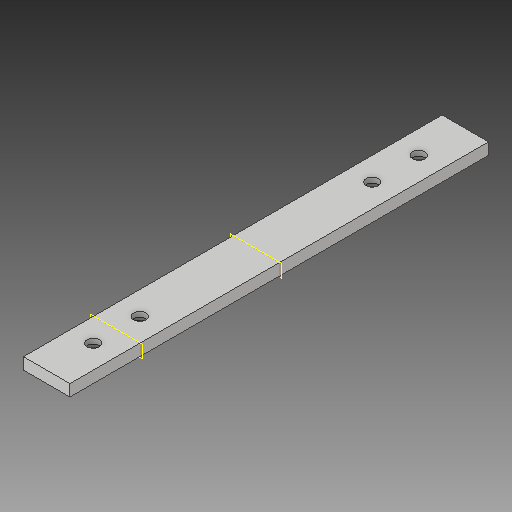
# Autodesk Inventor part: BandSawJigSupport
Saved by Autodesk Inventor 2019 (Build 230136000, 136)
## iProperties
Created: 2017-12-11
Part Number: BandSawJigSupport
Material: Generic
Document SubType Name: Modeling
Designer: steele
Density: 1 g/cm^3
Appearance: Default
Author: steele
Autodesk Inventor part; units mm, degrees
ref_plane "YZ Plane" through (0, 0, 0) normal (1, 0, 0) x (0, 1, 0)
ref_plane "XZ Plane" through (0, 0, 0) normal (0, 1, 0) x (-1, 0, 0)
sketch "Sketch1" plane through (0, 0, 0) normal (0, 1, 0) x (-1, 0, 0)
  line L0 (12.7, 114.3) -> (-12.7, 114.3)
  line L1 (-12.7, 114.3) -> (-12.7, -114.3)
  line L2 (-12.7, -114.3) -> (12.7, -114.3)
  line L3 (12.7, -114.3) -> (12.7, 114.3)
  line L4 (12.7, 114.3) -> (-12.7, -114.3) construction
  line L5 (-12.7, 114.3) -> (12.7, -114.3) construction
  point P0 (0, 0)
  dimension "d0" = 25.4
  dimension "d1" = 228.6
  constraints: 12 end point, 2 midpoint, 2 parallel, 1 horizontal, 1 perpendicular
  measures "d0" distance of L0.start L0.end
  measures "d1" distance of L1.end L0.end
extrude "Extrusion1" add sketch "Sketch1" against normal blind 6.35
sketch "Sketch3" plane through (0, -6.35, 0) normal (0, -1, 0) x (1, 0, 0)
  circle A0 centre (0, 63.5) radius 6.35
  line L0 (12.7, 114.3) -> (-12.7, 114.3) projected
  point P0 (0, 0)
  dimension "d5" = 12.7
  dimension "d6" = 50.8
  constraints: 1 centre point
  measures "d5" diameter of A0
  measures "d6" distance from line of L0 A0.centre
extrude "Extrusion2" cut sketch "Sketch3" against normal blind 3.556
sketch "Sketch4" plane through (0, -2.794, 63.5) normal (0, -1, 0) x (1, 0, 0)
  circle A0 centre (0, 0) radius 3.3782
  point P0 (0, -63.5)
  dimension "d9" = 6.7564
  constraints: 1 centre point
  measures "d9" diameter of A0
extrude "Extrusion3" cut sketch "Sketch4" against normal through all
ref_plane "Work Plane2" through (-12.7, 0, 76.2) normal (0, 0, 1) x (1, 0, 0)
mirror "Mirror1" about plane through (-12.7, 0, 76.2) normal (0, 0, 1) of "Extrusion3", "Extrusion2"
mirror "Mirror2" about plane through (0, 0, 0) normal (0, 0, 1) of "Extrusion3", "Extrusion2", "Mirror1"
body "Solid1"
